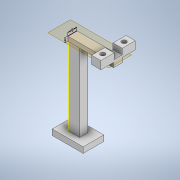
# Autodesk Inventor part: lobster training holder
Saved by Autodesk Inventor 2020.1 (Build 241239000, 239)
## iProperties
Created: 2019-07-30
Part Number: lobster training holder
Material: 일반
Document SubType Name: Modeling
Designer: Chang Ko
Mass: 7.19 g
Surface Area: 37.34 cm^2
Volume: 7.19 cm^3
Density: 1 g/cm^3
Appearance: 기본값
Author: Chang Ko
Autodesk Inventor part; units mm, degrees
ref_plane "YZ Plane" through (0, 0, 0) normal (1, 0, 0) x (0, 1, 0)
ref_plane "XZ Plane" through (0, 0, 0) normal (0, 1, 0) x (-1, 0, 0)
ref_plane "XY Plane" through (0, 0, 0) normal (0, 0, 1) x (1, 0, 0)
sketch "스케치1" plane through (0, 0, 0) normal (0, 1, 0) x (-1, 0, 0)
  line L0 (13.5, 9) -> (-13.5, 9)
  line L1 (-13.5, 9) -> (-13.5, -9)
  line L2 (-13.5, -9) -> (13.5, -9)
  line L3 (13.5, -9) -> (13.5, 9)
  point P0 (0, 0)
  dimension "d0" = 27
  dimension "d1" = 18
  dimension "d2" = 9
  dimension "d3" = 13.5
  constraints: 8 end point, 2 parallel, 1 horizontal, 1 perpendicular
  measures "d0" distance of L2.end L1.end
  measures "d1" distance of L1.end L0.end
  measures "d2" distance from line of point (0, 0) L0
  measures "d3" distance from line of L3 point (0, 0)
extrude "돌출1" add sketch "스케치1" along normal blind 5
sketch "스케치2" plane through (0, 5, 0) normal (0, 1, 0) x (1, 0, 0)
  line L0 (-5, -3.5) -> (5, -3.5)
  line L1 (5, -3.5) -> (5, 3.5)
  line L2 (5, 3.5) -> (-5, 3.5)
  line L3 (-5, 3.5) -> (-5, -3.5)
  line L4 (-13.5, -9) -> (13.5, -9) projected
  line L5 (-13.5, 9) -> (-13.5, -9) projected
  point P0 (0, 0)
  dimension "d6" = 10
  dimension "d7" = 7
  dimension "d8" = 5.5
  dimension "d9" = 8.5
  constraints: 8 end point, 1 horizontal, 1 parallel, 1 perpendicular, 1 vertical
  measures "d6" distance of L2.end L1.end
  measures "d7" distance of L1.end L0.end
  measures "d8" distance between parallel lines of L0 L4
  measures "d9" distance between parallel lines of L3 L5
extrude "돌출2" add sketch "스케치2" along normal blind 68
sketch "스케치12" plane through (-5, 5, -3.5) normal (-1, 0, 0) x (0, 0, 1)
  point P0 (3.5, -5)
sketch "스케치13" plane through (-5, 5, -3.5) normal (-1, 0, 0) x (0, 0, 1)
  line L0 (-0.5, 68) -> (7.5, 68)
  line L1 (7.5, 68) -> (7.5, 72)
  line L2 (7.5, 72) -> (-0.5, 72)
  line L3 (-0.5, 72) -> (-0.5, 68)
  line L4 (7, 68) -> (0, 68) projected
  line L5 (0, 0) -> (0, 68) projected
  line L6 (7, 0) -> (7, 68) projected
  point P0 (3.5, -5)
  point P1 (3.5, 68)
  point P2 (3.5, 72)
  dimension "d41" = 8
  dimension "d42" = 4
  constraints: 8 end point, 2 midpoint, 2 parallel, 1 collinear, 1 horizontal, 1 perpendicular
  measures "d41" distance of L2.end L1.end
  measures "d42" distance of L1.end L0.end
extrude "돌출5" add sketch "스케치13" against normal blind 40
ref_plane "작업 평면2" through (15, 77, -4) normal (0, 1, 0) x (1, 0, 0)
sketch "스케치14" plane through (15, 77, -4) normal (0, 1, 0) x (1, 0, 0)
  line L0 (20, -8) -> (20, 0) projected
  line L1 (20, -19.0746) -> (12, -19.0746)
  line L2 (12, -19.0746) -> (12, -0.5)
  line L3 (12, 10.9254) -> (20, 10.9254)
  line L4 (20, 10.9254) -> (20, 0)
  line L5 (-20, -8) -> (-20, 0) projected
  line L6 (-20, -8) -> (20, -8) projected
  line L7 (20, 0) -> (20, -8) projected
  line L8 (-20, 0) -> (20, 0)
  line L9 (12, -8) -> (12, -7.5)
  line L10 (12, 0) -> (12, 10.9254)
  line L11 (20, 0) -> (20, -0.5)
  line L12 (20, -8) -> (20, -19.0746)
  line L13 (12, -7.5) -> (20, -7.5)
  line L14 (20, -7.5) -> (20, -0.5)
  line L15 (20, -0.5) -> (12, -0.5)
  line L16 (12, -0.5) -> (12, -8)
  line L17 (20, 0) -> (20, -8) projected
  line L18 (12, -7.5) -> (12, -0.5)
  line L19 (12, -0.5) -> (12, 2.4254)
  line L20 (20, -7.5) -> (20, -8)
  line L21 (20, -0.5) -> (20, -7.5)
  point P0 (-15, -4)
  point P1 (20, -4)
  point P2 (20, -0.5)
  point P3 (20, 0)
  dimension "d46" = 8
  dimension "d47" = 30
  dimension "d50" = 7
  dimension "d67" = 0.5
  dimension "d68" = 0.5
  constraints: 35 end point, 29 parallel, 6 collinear, 6 perpendicular, 5 point on line, 2 horizontal, 1 midpoint
  measures "d46" distance of L3.start L3.end
  measures "d47" distance of L1.end L3.start
  measures "d50" distance of L11.end L13.end
  measures "d67" distance between parallel lines of L6 L13
  measures "d68" distance between parallel lines of L8 L15
extrude "돌출6" add sketch "스케치14" along normal blind 7 contours L6 L2 L13 L0 | L12 L1 L2 L6 | L15 L19 L8 L0 | L8 L10 L3 L4
extrude "돌출7" add sketch "스케치14" along normal blind 2 contours L13 L2 L15 L0
sketch "스케치16" plane through (15, 84, -4) normal (0, 1, 0) x (1, 0, 0)
  line L0 (12, -7.5) -> (12, -19.0746) projected
  line L1 (12, -19.0746) -> (20, -19.0746) projected
  line L2 (12, 10.9254) -> (12, -0.5) projected
  line L3 (20, 10.9254) -> (12, 10.9254) projected
  point P0 (-15, -4)
  point P1 (16, -13.3746)
  point P2 (16, 5.2254)
  dimension "d62" = 4
  dimension "d63" = 5.7
  dimension "d64" = 4
  dimension "d65" = 5.7
  measures "d62" distance from line of L0 point (16, -13.375)
  measures "d63" distance from line of L1 point (16, -13.375)
  measures "d64" distance from line of L2 point (16, 5.225)
  measures "d65" distance from line of L3 point (16, 5.225)
hole "구멍2" at (31, 84, 9.3746) at (31, 84, -9.2254) direction (0, -1, 0) diameter 4 depth 10.8 tip angle 118
